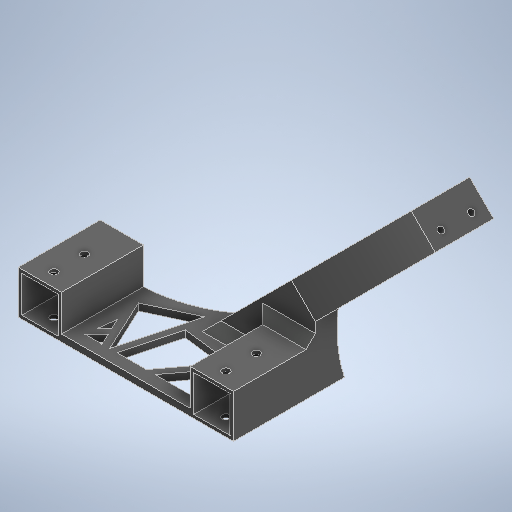
# Autodesk Inventor part: 45_deg_right
Saved by Autodesk Inventor 2026.1 (Build 301233020, 233B)
## iProperties
Created: 2026-02-01
Part Number: 45_deg_right
Material: 一般
Document SubType Name: Modeling
Designer: hibik
Density: 1 g/cm^3
Appearance: 既定
Author: hibik
Autodesk Inventor part; units mm, degrees
ref_plane "XZ Plane" through (0, 0, 0) normal (0, 1, 0) x (-1, 0, 0)
ref_plane "XY Plane" through (0, 0, 0) normal (0, 0, 1) x (1, 0, 0)
ref_plane "作業平面1" through (36.75, 0, 0) normal (1, 0, 0) x (0, 1, 0)
sketch "スケッチ1" plane through (0, 0, 0) normal (0, 0, 1) x (1, 0, 0)
  line L0 (36.75, 12.95) -> (36.75, -12.95) projected
  line L1 (29, -7.75) -> (44.5, -7.75)
  line L2 (44.5, -7.75) -> (44.5, 7.75)
  line L3 (44.5, 7.75) -> (29, 7.75)
  line L4 (29, 7.75) -> (29, -7.75)
  line L5 (29, -7.75) -> (44.5, 7.75) construction
  line L6 (44.5, -7.75) -> (29, 7.75) construction
  line L7 (46, -9.25) -> (27.5, -9.25)
  line L8 (27.5, -9.25) -> (27.5, 9.25)
  line L9 (27.5, 9.25) -> (46, 9.25)
  line L10 (46, 9.25) -> (46, -9.25)
  line L11 (46, -9.25) -> (27.5, 9.25) construction
  line L12 (27.5, -9.25) -> (46, 9.25) construction
  point P0 (0, 0)
  point P1 (36.75, 0)
  dimension "d1" = 15.5
  dimension "d2" = 1.5
  constraints: 24 end point, 5 midpoint, 4 parallel, 3 perpendicular, 2 horizontal, 1 horizontal alignment, 1 point on line
  measures "d1" distance of L2.end L3.end
  measures "d2" distance between parallel lines of L9 L3
extrude "押し出し1" add sketch "スケッチ1" along normal blind 25 contours L9 L10 L7 L0 L1 L2 L3 | L0 L3 L4 L1 L7 L8 L9
sketch "スケッチ2" plane through (27.5, 9.25, 0) normal (0, 1, 0) x (1, 0, 0)
  circle A0 centre (9.25, -19) radius 1.6
  line L0 (18.5, -25) -> (0, -25) projected
  circle A1 centre (9.25, -6) radius 1.6
  point P0 (-27.5, 0)
  point P1 (9.25, -25)
  dimension "d5" = 3.2
  dimension "d6" = 6
  dimension "d7" = 3.2
  dimension "d8" = 13
  constraints: 2 centre point, 2 vertical alignment, 1 midpoint
  measures "d5" diameter of A0
  measures "d6" distance from line of L0 A0.centre
  measures "d7" diameter of A1
  measures "d8" distance of A1.centre A0.centre
extrude "押し出し2" cut sketch "スケッチ2" against normal through all
ref_plane "作業平面2" through (27.5, 0, 0) normal (0, 1, 0) x (1, 0, 0)
mirror "ミラー1" about plane through (0, 0, 0) normal (1, 0, 0)
ref_plane "作業平面3" through (-27.5, -40, -9.25) normal (1, 0, 0) x (0, 0, -1)
ref_plane "作業平面4" through (-27.5, 1.5, 40) normal (0, 1, 0) x (1, 0, 0)
ref_plane "作業平面5" through (27.5, -14.25, 0) normal (0, -1, 0) x (1, 0, 0)
ref_plane "作業平面6" through (0, -14.25, 0) normal (0.7071068, -0.7071068, 0) x (0, 0, -1)
sketch "スケッチ10" plane through (0, -14.25, 0) normal (0.7071068, -0.7071068, 0) x (0, 0, -1)
  line L0 (40, 25.0763) -> (65, 25.0763)
  line L1 (65, 25.0763) -> (65, 15.0763)
  line L2 (65, 15.0763) -> (40, 15.0763)
  line L3 (40, 15.0763) -> (40, 25.0763)
  point P0 (0, 10.0763)
  point P1 (40, 20.0763)
  dimension "d78" = 25
  dimension "d79" = 10
  dimension "d81" = 40
  dimension "d90" = 10
  constraints: 8 end point, 2 parallel, 1 horizontal, 1 midpoint, 1 perpendicular
  measures "d78" distance of L1.end L2.end
  measures "d79" distance of L0.end L1.end
  measures "d81" distance from line of point (0, 10.076) L3
  measures "d90" vertical distance of point (0, 10.076) point (40, 20.076)
extrude "押し出し10" add sketch "スケッチ10" along normal blind 10
sketch "スケッチ11" plane through (17.7316, 3.4816, -65) normal (0.7071068, 0.7071068, 0) x (-0.7071068, 0.7071068, 0)
  circle A0 centre (-5, 19) radius 1.3
  circle A1 centre (-5, 6) radius 1.3
  line L0 (0, 25) -> (-10, 25) projected
  line L1 (0, 0) -> (-10, 0) projected
  point P0 (10.0763, 65)
  point P1 (-5, 25)
  point P2 (-5, 25)
  dimension "d84" = 6
  dimension "d85" = 6
  dimension "d86" = 2.6
  constraints: 2 centre point, 2 midpoint, 2 vertical alignment, 1 equal radius
  measures "d84" distance from line of L0 A0.centre
  measures "d85" distance from line of L1 A1.centre
  measures "d86" diameter of A0
extrude "押し出し11" cut sketch "スケッチ11" against normal through all
ref_plane "作業平面8" through (53.0869, 38.8369, -65) normal (0.7071068, 0.7071068, 0) x (-0.7071068, 0.7071068, 0)
sketch "スケッチ13" plane through (53.0869, 38.8369, -65) normal (0.7071068, 0.7071068, 0) x (-0.7071068, 0.7071068, 0)
  circle A0 centre (-5, 19) radius 1.3 projected
  circle A1 centre (-5, 6) radius 1.3 projected
  line L0 (0, 0) -> (0, 25) projected
  line L1 (0, 25) -> (-10, 25) projected
  line L2 (-10, 0) -> (-10, 25) projected
  line L3 (0, 0) -> (-10, 0) projected
  point P0 (10.0763, 65)
extrude "押し出し13" add sketch "スケッチ13" along normal blind 10
sketch "スケッチ14" plane through (0, -14.25, 0) normal (-0.7071068, 0.7071068, 0) x (-0.7071068, -0.7071068, 0)
  line L0 (-75.0763, -65) -> (-75.0763, -40) projected
  line L1 (-75.0763, -40) -> (-85.0763, -40) projected
  line L2 (-85.0763, -65) -> (-85.0763, -40) projected
  line L3 (-75.0763, -65) -> (-85.0763, -65) projected
  line L4 (-15.0763, -40) -> (-15.0763, -65) projected
  line L5 (-25.0763, -40) -> (-15.0763, -40) projected
  line L6 (-25.0763, -65) -> (-25.0763, -40) projected
  line L7 (-15.0763, -65) -> (-25.0763, -65) projected
  point P0 (-10.0763, 0)
extrude "押し出し14" add sketch "スケッチ14" along normal blind 3
sketch "スケッチ15" plane through (-2.1213, -12.1287, 0) normal (-0.7071068, 0.7071068, 0) x (0, 0, 1)
  line L0 (-40, 75.0763) -> (-40, 85.0763) projected
  line L1 (-65, 15.0763) -> (-65, 25.0763) projected
  line L2 (-40, 85.0763) -> (-65, 85.0763)
  line L3 (-65, 85.0763) -> (-65, 15.0763)
  line L4 (-65, 15.0763) -> (-40, 15.0763)
  line L5 (-40, 15.0763) -> (-40, 85.0763)
  point P0 (0, 10.0763)
  constraints: 8 end point, 2 parallel, 1 horizontal, 1 perpendicular
extrude "押し出し15" add sketch "スケッチ15" along normal blind 1.5
sketch "スケッチ16" plane through (-3.182, -11.068, 0) normal (-0.7071068, 0.7071068, 0) x (-0.7071068, -0.7071068, 0)
  circle A0 centre (-50.0763, -52.5) radius 37.1652
  line L0 (-85.0763, -40) -> (-85.0763, -65) projected
  line L1 (-15.0763, -40) -> (-85.0763, -40) projected
  circle A1 centre (-50.0763, -52.5) radius 33.1652
  point P0 (-10.0763, 0)
  point P1 (-85.0763, -52.5)
  point P2 (-50.0763, -40)
  point P3 (-80.7956, -40)
  point P4 (-19.3569, -40)
  point P5 (-15.0763, -40)
  dimension "d101" = 4
  constraints: 2 midpoint, 1 centre point, 1 coincident, 1 horizontal alignment, 1 vertical alignment, 3 other
extrude "押し出し16" add sketch "スケッチ16" against normal up to surface (14.5 mm away) contours L1 A1 A0
sketch "スケッチ17" plane through (0, 0, 0) normal (0, 0, -1) x (-1, 0, 0)
  line L0 (-46, -9.25) -> (-46, 9.25) projected
  line L1 (-27.5, -9.25) -> (-46, -9.25) projected
  line L2 (-27.5, 9.25) -> (-27.5, -9.25) projected
  line L3 (-46, 9.25) -> (-27.5, 9.25) projected
  line L4 (-44.5, -7.75) -> (-29, -7.75) projected
  line L5 (-44.5, 7.75) -> (-44.5, -7.75) projected
  line L6 (-29, 7.75) -> (-44.5, 7.75) projected
  line L7 (-29, -7.75) -> (-29, 7.75) projected
  line L8 (46, -9.25) -> (46, 9.25) projected
  line L9 (46, 9.25) -> (27.5, 9.25) projected
  line L10 (27.5, 9.25) -> (27.5, -9.25) projected
  line L11 (27.5, -9.25) -> (46, -9.25) projected
  line L12 (44.5, -7.75) -> (29, -7.75) projected
  line L13 (29, -7.75) -> (29, 7.75) projected
  line L14 (29, 7.75) -> (44.5, 7.75) projected
  line L15 (44.5, 7.75) -> (44.5, -7.75) projected
  point P0 (0, 0)
extrude "押し出し17" add sketch "スケッチ17" along normal blind 10
sketch "スケッチ18" plane through (27.5, -9.25, 25) normal (0, -1, 0) x (1, 0, 0)
  line L0 (-55, 0) -> (-55, -35) projected
  line L1 (18.5, -35) -> (0, -35) projected
  line L2 (-55, 0) -> (0, 0)
  line L3 (0, 0) -> (0, -35)
  line L4 (0, -35) -> (-55, -35)
  line L5 (-55, -35) -> (-55, 0)
  point P0 (-27.5, -25)
  constraints: 8 end point, 2 parallel, 1 horizontal, 1 perpendicular
extrude "押し出し18" add sketch "スケッチ18" against normal blind 3
sketch "スケッチ20" plane through (-3.182, -11.068, 0) normal (-0.7071068, 0.7071068, 0) x (-0.7071068, -0.7071068, 0)
  arc A0 (-15.0763, -40) -> (-85.0763, -40) centre (-50.0763, -52.5) ccw projected
  arc A1 (-19.3569, -40) -> (-80.7956, -40) centre (-50.0763, -52.5) ccw projected
  line L0 (-19.3569, -40) -> (-80.7956, -40) projected
  point P0 (-10.0763, 0)
sketch "スケッチ19" plane through (0, 0, -10) normal (0, 0, -1) x (-1, 0, 0)
  line L0 (-17.7316, -10.6605) -> (-67.2291, 38.8369) projected
  line L1 (-67.2291, 38.8369) -> (-56.976, 49.09) projected
  line L2 (-7.4786, -0.4075) -> (-56.976, 49.09) projected
  line L3 (-17.7316, -10.6605) -> (-7.4786, -0.4075) projected
  line L4 (-44.5, -7.75) -> (-44.5, 7.75) projected
  line L5 (-44.5, 7.75) -> (-29, 7.75) projected
  line L6 (-29, 7.75) -> (-29, -7.75) projected
  line L7 (-29, -7.75) -> (-44.5, -7.75) projected
  line L8 (46, 9.25) -> (27.5, 9.25) projected
  line L9 (27.5, 9.25) -> (27.5, -6.25) projected
  line L10 (-27.5, -6.25) -> (27.5, -6.25) projected
  line L11 (-27.5, -6.25) -> (-27.5, 9.25) projected
  line L12 (-27.5, 9.25) -> (-46, 9.25) projected
  line L13 (-46, 9.25) -> (-46, -9.25) projected
  line L14 (-46, -9.25) -> (46, -9.25) projected
  line L15 (46, -9.25) -> (46, 9.25) projected
  line L16 (44.5, -7.75) -> (29, -7.75) projected
  line L17 (29, -7.75) -> (29, 7.75) projected
  line L18 (29, 7.75) -> (44.5, 7.75) projected
  line L19 (44.5, 7.75) -> (44.5, -7.75) projected
  line L20 (-7.4786, -0.4075) -> (-1.636, -6.25)
  line L21 (-46, 9.25) -> (-46, 17.6079)
  line L22 (27.5, -6.25) -> (27.5, -9.25)
  point P0 (0, 0)
  constraints: 6 end point, 3 point on line, 1 collinear, 1 perpendicular, 1 vertical
extrude "押し出し19" add sketch "スケッチ19" along normal up to surface (30 mm away) contours L0 L1 L2 L3 L10 L11 L12 | L0 L12 L21 | L12 L11 L0 L6 L5 | L0 L5 L4 L7 L6 L11 L10 L14 L13 L12 | L5 L6 L0 | L0 L6 L7 L4 L5 | L20 L10 L3 | L0 L10 L11 | L0 L10 L3 L14 | L10 L22 L14 L3
sketch "スケッチ21" plane through (-3.182, -11.068, 0) normal (-0.7071068, 0.7071068, 0) x (-0.7071068, -0.7071068, 0)
  arc A0 (-15.0763, -40) -> (-85.0763, -40) centre (-50.0763, -52.5) ccw projected
  arc A1 (-19.3569, -40) -> (-80.7956, -40) centre (-50.0763, -52.5) ccw projected
  line L0 (-19.3569, -40) -> (-80.7956, -40) projected
  line L1 (-85.0763, -10) -> (-85.0763, -65) projected
  line L2 (-6.8137, -10) -> (-85.0763, -10) projected
  arc A2 (-55.0538, -10) -> (-85.0763, -40) centre (-38.429, -56.6598) ccw
  point P0 (-10.0763, 0)
  constraints: 2 point on circle, 1 centre point, 1 tangent
extrude "押し出し20" cut sketch "スケッチ21" against normal through all
sketch "スケッチ22" plane through (27.5, -6.25, 25) normal (0, 1, 0) x (1, 0, 0)
  line L0 (-25.864, 35) -> (-25.864, 65) projected
  arc A0 (-55, 35) -> (-25.864, 65) centre (-55, 64.1485) ccw
  line L1 (-73.5, 35) -> (-55, 35) projected
  line L2 (-55, 35) -> (-55, 65) projected
  line L3 (-55, 65) -> (-25.864, 65) projected
  point P0 (-27.5, 25)
  point P1 (-25.864, 63.297)
  constraints: 2 point on circle, 1 centre point, 1 tangent
extrude "押し出し21" cut sketch "スケッチ22" against normal through all contours A0 L2 L3 L0
sketch "スケッチ23" plane through (7.0711, -21.3211, 0) normal (0.7071068, -0.7071068, 0) x (-0.7071068, -0.7071068, 0)
  line L0 (-15.0763, 65) -> (-15.0763, 40) projected
  line L1 (15.9099, 10) -> (26.8701, 10) projected
  arc A0 (-15.0763, 40) -> (15.9099, 10) centre (15.9099, 41.0024) ccw
  ellipse E0 centre (15.9099, 39.1485) end of major axis (15.9099, 10) minor radius 20.6111 (-4.6924, 38.297) -> (15.9099, 10) ccw projected
  line L2 (-15.0763, 40) -> (-4.6924, 40) projected
  ellipse E1 centre (22.4506, -6) end of major axis (22.4506, -4.4) minor radius 1.1314 projected
  ellipse E2 centre (22.4506, -19) end of major axis (22.4506, -17.4) minor radius 1.1314 projected
  ellipse E3 centre (-29.5217, -19) end of major axis (-29.5217, -17.4) minor radius 1.1314 projected
  ellipse E4 centre (-29.5217, -6) end of major axis (-29.5217, -4.4) minor radius 1.1314 projected
  ellipse E5 centre (15.9099, 39.1485) end of major axis (15.9099, 10) minor radius 20.6111 (-4.6924, 38.297) -> (15.9099, 10) ccw projected
  line L3 (-4.6924, 38.297) -> (-4.6924, 40) projected
  line L4 (-15.0763, 40) -> (-4.6924, 40) projected
  arc A1 (-17.0711, 35.4147) -> (-15.0763, 40) centre (-50.0763, 52.5) ccw projected
  line L5 (-17.0711, 40) -> (-17.0711, 35.4147) projected
  line L6 (-19.3569, 40) -> (-17.0711, 40) projected
  arc A2 (-36.0624, 22.441) -> (-19.3569, 40) centre (-50.0763, 52.5) ccw projected
  line L7 (-36.0624, -25) -> (-36.0624, 22.441) projected
  line L8 (-36.0624, -25) -> (28.9914, -25) projected
  line L9 (28.9914, 10) -> (28.9914, -25) projected
  line L10 (15.9099, 10) -> (28.9914, 10) projected
  point P0 (-10.0763, 0)
  point P1 (-4.6924, 38.297)
  point P2 (-4.6924, 40)
  constraints: 2 point on circle, 1 centre point, 7 other
extrude "押し出し22" cut sketch "スケッチ23" against normal through all contours A0 L2 L3 E0
chamfer "面取り4" distance 4 angle 45 3 edges at (36.75, 9.25, -10) (27.5, 1.5, -10) (14.568, -6.25, -10)
fillet "フィレット1" radius 6 2 edges at (15.632, -2.5071, -40) (59.0757, 40.9366, -40)
sketch "スケッチ24" plane through (27.5, -6.25, 25) normal (0, 1, 0) x (1, 0, 0)
  line L0 (-5, 5) -> (-5, 25)
  line L1 (-5, 25) -> (-20, 5)
  line L2 (-20, 5) -> (-5, 5)
  line L3 (-8.4392, 25.4144) -> (-23.75, 5)
  line L4 (-23.75, 5) -> (-36.309, 5)
  line L5 (-36.309, 5) -> (-30.1385, 28.0287)
  line L6 (-30.1385, 28.0287) -> (-8.4392, 25.4144)
  line L7 (-39.4149, 5) -> (-30.864, 36.9125)
  line L8 (-30.864, 36.9125) -> (-50.1108, 27.9375)
  line L9 (-50.1108, 27.9375) -> (-39.4149, 5)
  line L10 (-42.725, 5) -> (-45.0386, 9.9614)
  line L11 (-45.0386, 9.9614) -> (-50, 5)
  line L12 (-50, 5) -> (-42.725, 5)
  line L13 (-49.4188, 9.8238) -> (-46.3878, 12.8549)
  line L14 (-46.3878, 12.8549) -> (-48.5063, 17.398)
  line L15 (-48.5063, 17.398) -> (-49.4188, 9.8238)
  line L16 (0, 31) -> (0, 0) projected
  line L17 (-55, 0) -> (0, 0) projected
  line L18 (-25.864, 31) -> (-25.864, 44.9125) projected
  line L19 (-55, 0) -> (-55, 35) projected
  point P0 (-27.5, 25)
  dimension "d120" = 5
  dimension "d121" = 5
  dimension "d122" = 20
  dimension "d123" = 3
  dimension "d124" = 15
  dimension "d125" = 60
  dimension "d126" = 5
  dimension "d127" = 8
  dimension "d128" = 75
  dimension "d129" = 3
  dimension "d130" = 3
  dimension "d131" = 5
  dimension "d132" = 3
  dimension "d133" = 50
  dimension "d134" = 45
  constraints: 32 end point, 6 point on line, 5 parallel, 3 perpendicular, 1 collinear, 1 horizontal, 1 vertical
  measures "d120" distance between parallel lines of L16 L0
  measures "d121" distance between parallel lines of L17 L2
  measures "d122" distance of L0.start L0.end
  measures "d123" distance between parallel lines of L3 L1
  measures "d124" distance of L1.end L0.start
  measures "d125" angle of L3 L6
  measures "d126" distance from line of L18 L7.end
  measures "d127" vertical distance of L18.end L7.end
  measures "d128" angle of L4 L5
  measures "d129" distance between parallel lines of L7 L5
  measures "d130" distance between parallel lines of L10 L9
  measures "d131" distance from line of L19 L11.end
  measures "d132" distance between parallel lines of L13 L11
  measures "d133" angle of L7 L8
  measures "d134" angle of L12 L11
extrude "押し出し23" cut sketch "スケッチ24" against normal through all
equation "\"d5\" = d7"
equation "\"d121\" = d120"
equation "\"d130\" = d129"
equation "\"d131\" = d120"
equation "\"d132\" = d130"
